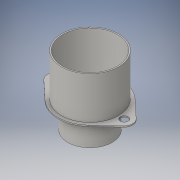
# Autodesk Inventor part: tube socket 9 pin
Saved by Autodesk Inventor 2016 (Build 200138000, 138)
## iProperties
Created: 2015-10-14
Part Number: tube socket 9 pin
Material: Generic
Document SubType Name: Modeling
Designer: jeremyhale
Density: 1 g/cm^3
Appearance: Default
Author: jeremyhale
Autodesk Inventor part; units mm, degrees
ref_plane "YZ Plane" through (0, 0, 0) normal (1, 0, 0) x (0, 1, 0)
ref_plane "XZ Plane" through (0, 0, 0) normal (0, 1, 0) x (-1, 0, 0)
ref_plane "XY Plane" through (0, 0, 0) normal (0, 0, 1) x (1, 0, 0)
sketch "Sketch1" plane through (0, 0, 0) normal (0, 1, 0) x (-1, 0, 0)
  line L0 (0, 0) -> (14.25, 0) construction
  circle A0 centre (14.25, 0) radius 1.65
  line L1 (0, 0) -> (17.75, 0) construction
  line L2 (17.75, 0) -> (17.75, -0.5019) construction
  line L3 (9.0658, 9.663) -> (16.6447, 2.5525)
  line L4 (9.0658, -9.663) -> (16.6447, -2.5525)
  arc A1 (16.6447, -2.5525) -> (16.6447, 2.5525) centre (14.25, 0) ccw
  line L5 (0, 0) -> (0, -5) construction
  circle A2 centre (-14.25, 0) radius 1.65
  line L6 (-9.0658, 9.663) -> (-16.6447, 2.5525)
  line L7 (-9.0658, -9.663) -> (-16.6447, -2.5525)
  arc A3 (-16.6447, 2.5525) -> (-16.6447, -2.5525) centre (-14.25, 0) ccw
  arc A4 (9.0658, 9.663) -> (-9.0658, 9.663) centre (0, 0) ccw
  arc A5 (-9.0658, -9.663) -> (9.0658, -9.663) centre (0, 0) ccw
  dimension "d1" = 14.25
  dimension "d2" = 3.3
  dimension "d3" = 17.75
  dimension "d7" = 13.25
  dimension "d8" = 5
  constraints: 16 end point, 8 point on circle, 8 symmetric about line, 6 centre point, 4 coincident, 3 tangent, 2 horizontal, 2 vertical, 2 other
  measures "d1" distance of L0.start L0.end
  measures "d2" diameter of A0
  measures "d3" distance of L0.start L1.end
  measures "d7" radius of A4
  measures "d8" distance of L0.start L5.end
extrude "Extrusion1" add sketch "Sketch1" along normal blind 0.5
sketch "Sketch2" plane through (0, 0.5, 0) normal (0, 1, 0) x (1, 0, 0)
  circle A0 centre (0, 0) radius 11.9
  circle A1 centre (0, 0) radius 11.4
  dimension "d11" = 23.8
  dimension "d12" = 22.8
  constraints: 2 centre point, 2 coincident
  measures "d11" diameter of A0
  measures "d12" diameter of A1
extrude "Extrusion2" add sketch "Sketch2" along normal blind 17.6
sketch "Sketch3" plane through (0, 0, 0) normal (0, -1, 0) x (1, 0, 0)
  circle A0 centre (0, 0) radius 9.25
  dimension "d15" = 18.5
  constraints: 1 centre point, 1 coincident
  measures "d15" diameter of A0
extrude "Extrusion3" add sketch "Sketch3" along normal blind 10.5
body "Solid1"
